Adaptador motor a arma (Autodesk Fusion 360 archive; units mm, degrees)
design "Modelo Motor Grande"
Autodesk Fusion 360 part; units mm, degrees
sketch "Boceto1" plane through (0, 0, 0) normal (0, 1, 0) x (1, 0, 0)
  circle A0 centre (0, 0) radius 54.5
  circle A1 centre (0, 0) radius 49
  circle A2 centre (0, 0) radius 24.5
  circle A3 centre (0, 0) radius 11.65
  line L0 (75, 0) -> (-75, 0) construction
  line L1 (54.5, -15) -> (54.5, 15) construction
  line L2 (-54.5, 15) -> (-54.5, -15) construction
  line L3 (-53.5747, 10) -> (-57.7, 10)
  line L4 (-62.8, 4.9) -> (-62.8, -4.9)
  line L5 (-57.7, -10) -> (-53.5747, -10)
  arc A4 (-57.7, 10) -> (-62.8, 4.9) centre (-57.7, 4.9) ccw
  arc A5 (-62.8, -4.9) -> (-57.7, -10) centre (-57.7, -4.9) ccw
  line L6 (-55.3641, 10) -> (-55.3641, 0) construction
  line L7 (-55.3641, -10) -> (-55.3641, 0) construction
  circle A6 centre (0, 0) radius 3.5
  line L8 (-2.4495, 2.5) -> (2.4495, 2.5)
  line L9 (-2.4495, -2.5) -> (2.4495, -2.5)
  line L10 (0, 2.5) -> (0, 3.5) construction
  line L11 (0, -2.5) -> (0, -3.5) construction
  circle A7 centre (0, 0) radius 2.5
  line L12 (53.5747, 10) -> (57.7, 10)
  line L13 (62.8, 4.9) -> (62.8, -4.9)
  line L14 (57.7, -10) -> (53.5747, -10)
  arc A8 (62.8, 4.9) -> (57.7, 10) centre (57.7, 4.9) ccw
  arc A9 (57.7, -10) -> (62.8, -4.9) centre (57.7, -4.9) ccw
  line L15 (55.8904, 10) -> (55.8904, 0) construction
  line L16 (55.8904, 0) -> (55.8904, -10) construction
  circle A10 centre (0, 0) radius 46.5
  circle A11 centre (0, 0) radius 8.75
  circle A12 centre (-57.3, -4.5) radius 3.5
  circle A13 centre (57.3, 4.5) radius 3.5
  line L17 (57.7, 4.9) -> (57.7, -4.9) construction
  line L18 (-57.7, 4.9) -> (-57.7, -4.9) construction
  line L19 (57.3, 4.5) -> (60.8, 4.5) construction
  line L20 (60.8, 4.5) -> (62.8, 4.5) construction
  line L21 (-57.3, -4.5) -> (-60.8, -4.5) construction
  line L22 (-60.8, -4.5) -> (-62.8, -4.5) construction
  line L23 (57.3, 4.5) -> (57.3, 8) construction
  line L24 (57.3, 8) -> (57.3, 10) construction
  line L25 (-57.3, -4.5) -> (-57.3, -8) construction
  line L26 (-57.3, -8) -> (-57.3, -10) construction
  line L27 (0, 75) -> (0, -75) construction
  line L28 (57.3, 4.5) -> (0, 4.5) construction
  line L29 (-57.3, -4.5) -> (0, -4.5) construction
  line L30 (-57.3, -4.5) -> (-57.3, 0) construction
  line L31 (57.3, 4.5) -> (57.3, 0) construction
  dimension "d1" = 109
  dimension "d2" = 98
  dimension "d3" = 49
  dimension "d4" = 23.3
  dimension "d7" = 5.1
  dimension "d8" = 5.1
  dimension "d9" = 9.8
  dimension "d12" = 7
  dimension "d13" = 5
  dimension "d14" = 5.1
  dimension "d15" = 5.1
  dimension "d18" = 9.8
  dimension "d19" = 93
  dimension "d20" = 17.5
  dimension "d21" = 7
  dimension "d22" = 7
  dimension "d115" = 9
  dimension "d116" = 2
  dimension "d117" = 2
  dimension "d118" = 2
  dimension "d119" = 2
  dimension "d120" = 114.6
  dimension "d121" = 20
  dimension "d122" = 20
  constraint coincident A0.centre A1.centre
  constraint concentric A0 A1
  constraint concentric A1 A3
  constraint horizontal L0
  constraint coincident A0.centre L0
  constraint midpoint A0.centre L0
  constraint perpendicular L0 L1
  constraint perpendicular L0 L2
  constraint tangent A0 L1
  constraint tangent A0 L2
  constraint coincident A0 L3.start
  constraint perpendicular L2 L3
  constraint perpendicular L0 L4
  constraint coincident A0 L5.end
  constraint perpendicular L2 L5
  constraint tangent L3 A4
  constraint tangent L4 A4
  constraint tangent L4 A5
  constraint tangent L5 A5
  constraint coincident L3 L6.start
  constraint perpendicular L3 L6
  constraint coincident L5 L7.start
  constraint perpendicular L0 L7
  constraint equal L6 L7
  constraint coincident L0 L6.end
  constraint concentric A0 A6
  constraint coincident A6 L8.start
  constraint coincident A6 L8.end
  constraint horizontal L8
  constraint coincident A6 L9.start
  constraint coincident A6 L9.end
  constraint parallel L8 L9
  constraint midpoint L8 L10.start
  constraint coincident A6 L10.end
  constraint perpendicular L8 L10
  constraint midpoint L9 L11.start
  constraint perpendicular L9 L11
  constraint equal L10 L11
  constraint coincident A6 L11.end
  constraint concentric A6 A7
  constraint coincident L10.start A7
  constraint coincident A0 L12.start
  constraint perpendicular L1 L12
  constraint perpendicular L0 L13
  constraint coincident A0 L14.end
  constraint perpendicular L13 L14
  constraint tangent L12 A8
  constraint tangent L13 A8
  constraint tangent L13 A9
  constraint tangent L14 A9
  constraint coincident L12 L15.start
  constraint coincident L0 L15.end
  constraint perpendicular L0 L15
  constraint coincident L14 L16.end
  constraint perpendicular L14 L16
  constraint equal L15 L16
  constraint concentric A0 A10
  constraint concentric A2 A11
  constraint coincident A8.centre L17.start
  constraint coincident A9.centre L17.end
  constraint coincident A4.centre L18.start
  constraint coincident A5.centre L18.end
  constraint coincident A13.centre L19.start
  constraint perpendicular L17 L19
  constraint coincident L13 L20.end
  constraint perpendicular L13 L20
  constraint coincident A13 L19.end
  constraint coincident A12.centre L21.start
  constraint coincident A12 L21.end
  constraint perpendicular L18 L21
  constraint coincident L4 L22.end
  constraint perpendicular L4 L22
  constraint coincident A13 L23.end
  constraint perpendicular L19 L23
  constraint coincident L12 L24.end
  constraint perpendicular L12 L24
  constraint coincident A12 L25.end
  constraint perpendicular L21 L25
  constraint coincident L5 L26.end
  constraint perpendicular L5 L26
  constraint vertical L27
  constraint midpoint A0.centre L27
  constraint coincident L27 L28.end
  constraint perpendicular L27 L28
  constraint coincident L27 L29.end
  constraint perpendicular L27 L29
  constraint equal L28 L29
  constraint coincident L0 L30.end
  constraint perpendicular L0 L30
  constraint coincident L0 L31.end
  constraint perpendicular L0 L31
  constraint equal L30 L31
  measures "d1" diameter of A0
  measures "d2" diameter of A1
  measures "d3" diameter of A2
  measures "d4" diameter of A3
  measures "d7" radius of A4
  measures "d8" radius of A5
  measures "d9" distance of L4.start L4.end
  measures "d12" diameter of A6
  measures "d13" distance of L8 L9
  measures "d14" radius of A8
  measures "d15" radius of A9
  measures "d18" distance of L13.start L13.end
  measures "d19" diameter of A10
  measures "d20" diameter of A11
  measures "d21" diameter of A12
  measures "d22" diameter of A13
  measures "d115" vertical distance of A12.centre A13.centre
  measures "d116" distance of L19.end L20.end
  measures "d117" distance of L21.end L22.end
  measures "d118" distance of L25.end L26.end
  measures "d119" distance of L23.end L24.end
  measures "d120" horizontal distance of A12.centre A13.centre
  measures "d121" distance of L12 L14
  measures "d122" distance of L3 L5
extrude "Extruir1" add sketch "Boceto1" along normal blind 2.5 contours A0 A12 A13 | A0 L12 L13 L14 A8 A9 A13 | A0 L3 L4 L5 A4 A5 A12 makes body 1
extrude "Extruir2" add sketch "Boceto1" along normal blind 16 contours A1 | A2 | A3 | A6 L8 L9 A7 | A6 L8 | A6 L9 | A6 L8 L9 A7 | A7 | A10 | A11 bodies 1
extrude "Extruir3" add sketch "Boceto1" along normal blind 17 contours A1 bodies 1
extrude "Extruir4" add sketch "Boceto1" along normal blind 19.9 contours A2 | A3 | A6 L8 L9 A7 | A6 L8 | A6 L9 | A6 L8 L9 A7 | A7 | A11 bodies 1
extrude "Extruir5" add sketch "Boceto1" along normal blind 25.9 contours A6 L8 L9 A7 | A6 L8 | A6 L9 | A6 L8 L9 A7 | A7 | A11 bodies 1
extrude "Extruir6" add sketch "Boceto1" along normal blind 27.9 contours A3 bodies 1
extrude "Extruir7" add sketch "Boceto1" along normal blind 28.9 contours A6 L8 L9 A7 | A6 L8 | A6 L9 | A6 L8 L9 A7 | A7 bodies 1
extrude "Extruir8" add sketch "Boceto1" along normal blind 39.9 contours A6 L8 L9 A7 | A6 L8 L9 A7 | A7 bodies 1
extrude "Extruir9" add sketch "Boceto1" along normal blind 46.2 contours A7 bodies 1
sketch "Boceto2" plane through (0, 0, 0) normal (0, 1, 0) x (1, 0, 0)
  circle A0 centre (0, 0) radius 54.5
  circle A1 centre (0, 0) radius 49
  circle A2 centre (0, 0) radius 46.5
  circle A3 centre (0, 0) radius 27.5
  circle A4 centre (0, 0) radius 11.7
  line L0 (0, 0) -> (-7.3109, 26.5104) construction
  line L1 (-4.7254, 17.135) -> (-1.1103, 18.1319)
  line L2 (-0.0631, 19.9767) -> (-0.8606, 22.8688)
  line L3 (-2.7054, 23.916) -> (-6.3205, 22.9191)
  line L4 (-6.3205, 22.9191) -> (-9.9355, 21.9222)
  line L5 (-10.9828, 20.0774) -> (-10.1852, 17.1853)
  line L6 (-8.3404, 16.1381) -> (-4.7254, 17.135)
  arc A5 (-10.1852, 17.1853) -> (-8.3404, 16.1381) centre (-8.7392, 17.5841) ccw
  arc A6 (-9.9355, 21.9222) -> (-10.9828, 20.0774) centre (-9.5368, 20.4761) ccw
  arc A7 (-1.1103, 18.1319) -> (-0.0631, 19.9767) centre (-1.5091, 19.578) ccw
  arc A8 (-0.8606, 22.8688) -> (-2.7054, 23.916) centre (-2.3066, 22.47) ccw
  line L7 (-1.5091, 19.578) -> (-2.3066, 22.47) construction
  line L8 (-9.5368, 20.4761) -> (-8.7392, 17.5841) construction
  line L9 (-9.138, 19.0301) -> (-1.9079, 21.024) construction
  circle A9 centre (-7.692, 19.4289) radius 1.5 construction
  circle A10 centre (-3.3539, 20.6252) radius 1.5 construction
  line L10 (0, 0) -> (-27.4121, 2.1971) construction
  line L11 (0, 0) -> (22.4112, 15.9371) construction
  circle A11 centre (-19, 1.5229) radius 2.5
  circle A12 centre (15.4841, 11.0111) radius 2.5
  dimension "d41" = 55
  dimension "d42" = 23.4
  dimension "d43" = 1.5
  dimension "d44" = 1.5
  dimension "d45" = 1.5
  dimension "d46" = 1.5
  dimension "d47" = 3
  dimension "d48" = 3
  dimension "d49" = 3
  dimension "d50" = 3
  dimension "d51" = 3
  dimension "d52" = 7.5
  dimension "d53" = 70
  dimension "d54" = 70
  dimension "d55" = 5
  dimension "d56" = 5
  dimension "d57" = 19
  dimension "d58" = 19
  dimension "d125" = 6
  dimension "d126" = 10.5
  constraint concentric A2 A3
  constraint concentric A2 A4
  constraint coincident A0.centre A1.centre
  constraint coincident A3 L0.end
  constraint coincident L0 L1.start
  constraint perpendicular L0 L1
  constraint perpendicular L1 L2
  constraint coincident L0 L3.end
  constraint perpendicular L0 L3
  constraint perpendicular L0 L4
  constraint perpendicular L3 L5
  constraint perpendicular L0 L6
  constraint coincident L1.start L6.end
  constraint tangent L5 A5
  constraint tangent L6 A5
  constraint tangent L4 A6
  constraint tangent L5 A6
  constraint tangent L1 A7
  constraint tangent L2 A7
  constraint tangent L2 A8
  constraint tangent L3 A8
  constraint equal L3 L4
  constraint coincident A7.centre L7.start
  constraint coincident A8.centre L7.end
  constraint coincident A6.centre L8.start
  constraint coincident A5.centre L8.end
  constraint midpoint L8 L9.start
  constraint midpoint L7 L9.end
  constraint coincident L9 A9.centre
  constraint coincident L9 A10.centre
  constraint coincident A3 L10.end
  constraint coincident A3 L11.end
  constraint coincident L10 A11.centre
  constraint coincident L11 A12.centre
  measures "d41" diameter of A3
  measures "d42" diameter of A4
  measures "d43" radius of A5
  measures "d44" radius of A6
  measures "d45" radius of A7
  measures "d46" radius of A8
  measures "d47" diameter of A9
  measures "d48" diameter of A10
  measures "d49" distance of L5 A9.centre
  measures "d50" distance of L2 A10.centre
  measures "d51" distance of L1 A10.centre
  measures "d52" distance of L7 L8
  measures "d53" angle of A0.centre L0.end L10.end
  measures "d54" angle of A0.centre L0.end L11.end
  measures "d55" diameter of A11
  measures "d56" diameter of A12
  measures "d57" horizontal distance of A0.centre A11.centre
  measures "d58" distance of A0.centre A12.centre
  measures "d125" distance of L4 L6
  measures "d126" distance of L2 L5
extrude "Extruir10" cut sketch "Boceto2" along normal blind 1 contours A1 bodies 1
extrude "Extruir11" add sketch "Boceto2" against normal blind 2.9 contours A3 | A4 | L1 L2 L3 L4 L5 L6 A5 A6 A7 A8 | A11 | A12 bodies 1
extrude "Extruir12" add sketch "Boceto2" against normal blind 11.9 contours A4 bodies 1
extrude "Extruir13" add sketch "Boceto2" against normal blind 3.9 contours A11 | A12 bodies 1
extrude "Extruir14" add sketch "Boceto2" against normal blind 7.4 contours L1 L2 L3 L4 L5 L6 A5 A6 A7 A8 bodies 1
fillet "Empalme1" radius 7 1 edges at (-53.5747, 1.25, 10) on bodies 1
fillet "Empalme1" radius 7 1 edges at (53.5747, 1.25, 10) on bodies 1
fillet "Empalme1" radius 7 1 edges at (53.5747, 1.25, -10) on bodies 1
fillet "Empalme1" radius 7 1 edges at (-53.5747, 1.25, -10) on bodies 1
fillet "Empalme2" radius 3 2 edges at (-22.842, 16, -8.8596) (-22.842, 19.9, 8.8596) on bodies 1
fillet "Empalme3" radius 1.2 2 edges at (-45.684, 17, 17.7192) (-43.3532, 17, -16.8151) on bodies 1
fillet "Empalme4" radius 3 1 edges at (-45.684, 2.5, -17.7192) on bodies 1
fillet "Empalme5" radius 3 1 edges at (-25.639, -2.9, -9.9444) on bodies 1
fillet "Empalme6" radius 4.5 curvature continuous tangency weight 2 1 edges at (-10.9082, -11.9, -4.2309) on bodies 1
fillet "Empalme7" radius 1.5 8 edges at (-1.5661, -7.4, -23.7745) (-0.4619, -7.4, -21.4228) (-0.2046, -7.4, -18.8374) (-4.7254, -7.4, -17.135) (-9.4797, -7.4, -16.2796) (-10.584, -7.4, -18.6313) (-10.8412, -7.4, -21.2166) (-6.3205, -7.4, -22.9191) on bodies 1
fillet "Empalme8" radius 0.5 tangency weight 1.75 2 edges at (-21.3308, -3.9, -2.4269) (13.1533, -3.9, -11.9151) on bodies 1
fillet "Empalme9" radius 1.2 1 faces at (47.8111, 1, 4.7445) on bodies 1
fillet "Empalme10" radius 1.3 2 edges at (-45.684, 0, 17.7192) (-43.3532, 0, -16.8151) on bodies 1
fillet "Empalme11" radius 1.3 1 edges at (-43.3532, 16, 16.8151) on bodies 1
fillet "Empalme12" radius 3 1 edges at (-10.8616, 19.9, -4.2128) on bodies 1
fillet "Empalme14" radius 3 1 edges at (-10.9082, -2.9, 4.2309) on bodies 1
fillet "Empalme13" radius 1.35 tangency weight 0.5 1 edges at (-10.8616, 27.9, 4.2128) on bodies 1
thread "Rosca1" "ISO Metric profile 5.0 M5x0.8 6g" major diameter 4.901 minor diameter 3.9895 pitch 0.8 angle 60 modelled right hand crest width 0.1157 on face at (-1.5587, 42, -1.9546) from (0, 41.2, 0) to (0, 46.2, 0) crest through (2.4505, 39.7, 0) on bodies 1
hole "Agujero1" at (0, 25.9, 0) direction (0, 1, 0) diameter 22 depth 1.25 tip angle 180 bodies 1 makes body 2 at (-2.7179, 31.9833, -2.2053)
extrude "Extruir15" add 1 faces at (1.7551, 27.15, 0.0926) along direction (0, -1, 0) blind 1.5 on bodies 2 bodies 2 1
split "Dividir1" by face at (-2.7179, 31.5667, -2.2053) of body 2 bodies 2 makes body 3 at (24.4689, 0, -31.0915)
split "Dividir2" by plane through (0, 25.9, 0) normal (0, 1, 0) bodies 2 makes body 4 at (-2.7179, 31.5667, -2.2053)
combine "Combinar1" operation add target body 2 tool bodies 3
copy_body "Cuerpo - > Comp.1" bodies 4 removing the originals makes body 5 in component "Driveshaft"
copy_body "Cuerpo - > Comp.2" bodies 2 removing the originals makes body 6 in component "Cuerpo Motor"
component "Driveshaft" placed x (1, 0, 0) y (0, 1, 0) z (0, 0, 1) at (0, 0, 0)
component "Cuerpo Motor" placed x (1, 0, 0) y (0, 1, 0) z (0, 0, 1) at (0, 0, 0)
equation "d7 = d8"
equation "d14 = d15"
equation "d19 = d2 - 5 mm"
equation "d29 = 17 mm + 2.9 mm"
equation "d31 = 17 mm + 2.9 mm + 6 mm"
equation "d33 = 17 mm + 2.9 mm + 8 mm"
equation "d35 = 27.90 mm + 1 mm"
equation "d37 = 28.90 mm + 11 mm"
equation "d39 = 39.90 mm + 6.3 mm"
equation "d44 = d43"
equation "d45 = d43"
equation "d46 = d43"
equation "d48 = d47"
equation "d49 = d47"
equation "d50 = d49"
equation "d51 = d49"
equation "d52 = d47 + d48 + d47 / 2"
equation "d54 = d53"
equation "d56 = d55"
equation "d58 = d57"
equation "d63 = -2.90 mm - 8 mm - 1 mm"
equation "d67 = -2.90 mm - 4.5 mm"
equation "d105 = 24.5 mm - 2.5 mm"
equation "d115 = 16 mm - 7 mm"
named bodies: "Cuerpo Motor", "Driveshaft"

design "helice" references "Adaptador"
Autodesk Fusion 360 part; units mm, degrees
sketch "Boceto1" plane through (0, 0, 0) normal (0, 0, 1) x (1, 0, 0)
  line L0 (20, 75) -> (-20, 75)
  line L1 (-20, 75) -> (-20, -75)
  line L2 (-20, -75) -> (20, -75)
  line L3 (20, -75) -> (20, 75)
  line L4 (20, 75) -> (-20, -75) construction
  line L5 (-20, 75) -> (20, -75) construction
  circle A0 centre (0, 0) radius 1.25
  dimension "d1" = 40
  dimension "d2" = 150
  dimension "d5" = 2.5
  constraint horizontal L0
  constraint perpendicular L0 L1
  constraint parallel L0 L2
  constraint parallel L1 L3
  constraint coincident L4 A0.centre
  constraint coincident L5 A0.centre
  constraint coincident A0.centre origin
  measures "d1" distance of L1.end L2.end
  measures "d2" distance of L0.end L1.end
  measures "d5" diameter of A0
extrude "Extruir2" add sketch "Boceto1" along normal blind 3.3
sketch "Boceto2" plane through (0, 0, 0) normal (0, 0, -1) x (-1, 0, 0)
  circle A0 centre (0, 0) radius 1.25
  line L0 (-20, 75) -> (-20, -75)
  line L1 (-20, -75) -> (20, -75)
  line L2 (20, -75) -> (20, 75)
  line L3 (20, 75) -> (-20, 75)
  circle A1 centre (-5.889, -3.4) radius 1.5
  circle A2 centre (0, -6.8) radius 1.5
  circle A3 centre (5.889, -3.4) radius 1.5
  circle A4 centre (5.889, 3.4) radius 1.5
  circle A5 centre (0, 6.8) radius 1.5
  arc A6 (0, -2.6) -> (0, 2.6) centre (0, 0) ccw construction
  arc A7 (0, 2.6) -> (0, -2.6) centre (0, 0) ccw construction
  circle A8 centre (-5.889, 3.4) radius 1.5
  circle A9 centre (0, 0) radius 4.1
  dimension "d8" = 2.6
  dimension "d9" = 8.2
  constraint concentric A6 A9
  measures "d8" radius of A6
  measures "d9" diameter of A9
extrude "Extruir3" cut sketch "Boceto2" against normal blind 10 contours A1 | A2 | A3 | A4 | A5 | A8 | A9
move_body "Desplazar1" bodies 1 to x (0, -1, 0) y (1, 0, 0) z (0, 0, 1) at (0, 0, 0)
extrude "Extruir4" cut sketch "Boceto2" against normal blind 10 contours A1 | A2 | A3 | A4 | A5 | A8
move_body "Desplazar2" bodies 1 to x (0, 1, 0) y (-1, 0, 0) z (0, 0, 1) at (0, 0, 0)
extrude "Extruir5" add 1 faces at (-6.6667, -75, 2.2) along direction (0, -1, 0) blind 40
extrude "Extruir6" add 1 faces at (6.6667, 75, 2.2) along direction (0, 1, 0) blind 40
equation "d9 = d8 * 2 + 3 mm"
